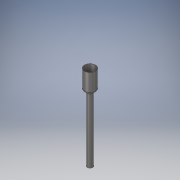
# Autodesk Inventor part: still pipe standin
Saved by Autodesk Inventor 2018 (Build 220112000, 112)
## iProperties
Created: 2018-10-16
Part Number: still pipe standin
Material: Stainless Steel, Austenitic
Document SubType Name: Modeling
Designer: freyja
Density: 8 g/cm^3
Appearance: Semi-Polished
Author: freyja
Autodesk Inventor part; units mm, degrees
ref_plane "YZ Plane" through (0, 0, 0) normal (1, 0, 0) x (0, 1, 0)
ref_plane "XZ Plane" through (0, 0, 0) normal (0, 1, 0) x (-1, 0, 0)
ref_plane "XY Plane" through (0, 0, 0) normal (0, 0, 1) x (1, 0, 0)
sketch "Sketch1" plane through (0, 0, 0) normal (0, 1, 0) x (-1, 0, 0)
  circle A0 centre (0, 0) radius 12.5
  circle A1 centre (0, 0) radius 12.192
  dimension "d0" = 25
  dimension "d1" = 24.384
  constraints: 2 centre point, 2 coincident
  measures "d0" diameter of A0
  measures "d1" diameter of A1
extrude "Extrusion1" add sketch "Sketch1" along normal blind 304.8
sketch "Sketch2" plane through (0, 304.8, 0) normal (0, 1, 0) x (1, 0, 0)
  circle A0 centre (0, 0) radius 24.765
  circle A1 centre (0, 0) radius 25.4
  dimension "d4" = 50.8
  dimension "d5" = 49.53
  constraints: 2 centre point, 2 coincident
  measures "d4" diameter of A1
  measures "d5" diameter of A0
extrude "Extrusion2" add sketch "Sketch2" along normal blind 304.8
sketch "Sketch3" plane through (0, 304.8, 0) normal (0, -1, 0) x (1, 0, 0)
  circle A0 centre (0, 0) radius 25.4
  circle A1 centre (0, 0) radius 12.192
  dimension "d8" = 50.8
  dimension "d12" = 24.384
  constraints: 2 centre point, 2 coincident
  measures "d8" diameter of A0
  measures "d12" diameter of A1
extrude "Extrusion3" add sketch "Sketch3" against normal blind 1.27
fillet "Fillet1" radius 7.874 3 edges at (12.5, 304.8, 0) (-24.765, 306.07, 0) (-25.4, 304.8, 0)
fillet "Fillet2" radius 7.874 1 edges at (-12.192, 306.07, 0)
body "Solid1"
